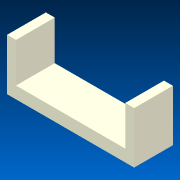
# Autodesk Inventor part: Rear B Spacer
Saved by Autodesk Inventor 2012 (Build 160160000, 160)
## iProperties
Created: 2012-07-06
Part Number: Rear B Spacer
Material: Default
Document SubType Name: Modeling
Designer: Hemant
Density: 1 g/cm^3
Author: Hemant
Autodesk Inventor part; units mm, degrees
ref_plane "YZ Plane" through (0, 0, 0) normal (1, 0, 0) x (0, 1, 0)
ref_plane "XZ Plane" through (0, 0, 0) normal (0, 1, 0) x (-1, 0, 0)
ref_plane "XY Plane" through (0, 0, 0) normal (0, 0, 1) x (1, 0, 0)
sketch "Sketch1" plane through (0, 0, 0) normal (0, 0, 1) x (1, 0, 0)
  line L0 (0, 0) -> (-58.42, 0)
  line L1 (-58.42, 0) -> (-58.42, -337.82)
  line L2 (-58.42, -337.82) -> (774.7, -337.82)
  line L3 (774.7, -337.82) -> (774.7, 0)
  line L4 (774.7, 0) -> (716.28, 0)
  line L5 (716.28, 0) -> (716.28, -259.08)
  line L6 (716.28, -259.08) -> (0, -259.08)
  line L7 (0, 0) -> (0, -259.08)
  dimension "d0" = 58.42
  dimension "d1" = 337.82
  dimension "d2" = 337.82
  dimension "d3" = 58.42
  dimension "d4" = 78.74
  dimension "d5" = 833.12
  constraints: 16 end point, 5 perpendicular, 2 parallel, 1 horizontal
  measures "d0" distance of L0.start L0.end
  measures "d1" distance of L0.end L1.end
  measures "d2" distance of L2.end L3.end
  measures "d3" distance of L3.end L4.end
  measures "d4" distance between parallel lines of L2 L6
  measures "d5" distance of L1.end L2.end
extrude "Extrusion1" add sketch "Sketch1" along normal blind 254
body "Solid1"
